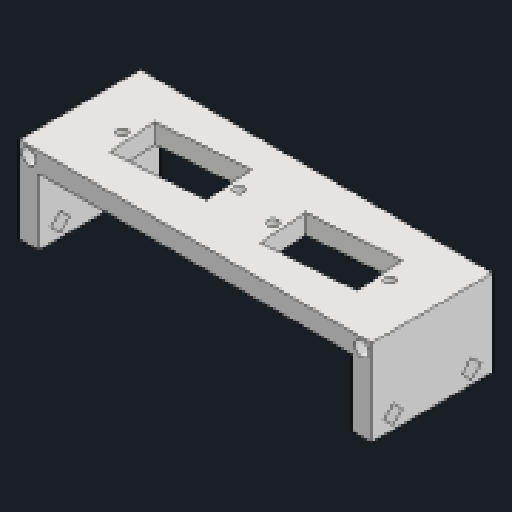
# Autodesk Inventor part: Module Frame
Saved by Autodesk Inventor 2023.2 (Build 272271030, 271C)
## iProperties
Created: 2024-02-26
Part Number: Module Frame
Material: Generic
Document SubType Name: Modeling
Designer: robpl
Density: 1 g/cm^3
Appearance: Default
Author: robpl
Autodesk Inventor part; units mm, degrees
ref_plane "YZ Plane" through (0, 0, 0) normal (1, 0, 0) x (0, 1, 0)
ref_plane "XZ Plane" through (0, 0, 0) normal (0, 1, 0) x (-1, 0, 0)
ref_plane "XY Plane" through (0, 0, 0) normal (0, 0, 1) x (1, 0, 0)
sketch "Sketch1" plane through (0, 0, 0) normal (0, 0, 1) x (1, 0, 0)
  line L0 (-40, 0) -> (40, 0)
  line L1 (40, 0) -> (40, 5)
  line L2 (40, 5) -> (-40, 5)
  line L3 (-40, 5) -> (-40, 0)
  line L4 (-40, 5) -> (-45, 5)
  line L5 (-45, 5) -> (-45, -17)
  line L6 (-45, -17) -> (-40, -17)
  line L7 (-40, -17) -> (-40, 5)
  line L8 (40, 5) -> (45, 5)
  line L9 (45, 5) -> (45, -17)
  line L10 (45, -17) -> (40, -17)
  line L11 (40, -17) -> (40, 5)
  point P0 (0, 0)
  point P1 (0, 0)
  point P2 (40, 0)
  dimension "d0" = 5
  dimension "d1" = 80
  dimension "d2" = 22
  dimension "d11" = 5
  constraints: 24 end point, 6 parallel, 3 horizontal, 3 perpendicular, 2 equal length, 1 coincident, 1 midpoint
  measures "d0" distance of L0.end L1.end
  measures "d1" distance of L0.start L0.end
  measures "d2" distance of L6.end L2.end
  measures "d11" distance of L9.end L10.end
extrude "Extrusion1" add sketch "Sketch1" along normal mid plane 31
sketch "Sketch2" plane through (45, -17, -15.5) normal (1, 0, 0) x (0, 0, -1)
  line L0 (-27.9042, 3.5) -> (-25.5, 1.0958)
  line L1 (-25.5, 1.0958) -> (-23.0958, 3.5)
  line L2 (-23.0958, 3.5) -> (-25.5, 5.9042)
  line L3 (-25.5, 5.9042) -> (-27.9042, 3.5)
  line L4 (-27.9042, 3.5) -> (-23.0958, 3.5) construction
  line L5 (-25.5, 1.0958) -> (-25.5, 5.9042) construction
  line L6 (-7.9042, 3.5) -> (-5.5, 1.0958)
  line L7 (-5.5, 1.0958) -> (-3.0958, 3.5)
  line L8 (-3.0958, 3.5) -> (-5.5, 5.9042)
  line L9 (-5.5, 5.9042) -> (-7.9042, 3.5)
  line L10 (-7.9042, 3.5) -> (-3.0958, 3.5) construction
  line L11 (-5.5, 1.0958) -> (-5.5, 5.9042) construction
  line L12 (0, 22) -> (-31, 22) projected
  point P0 (-15.5, 17)
  point P1 (-25.5, 3.5)
  point P2 (-5.5, 3.5)
  point P3 (-5.5, 3.5)
  point P4 (-25.5, 3.5)
  point P5 (-5.5, 3.5)
  point P6 (-15.5, 22)
  point P7 (-25.5, 3.5)
  dimension "d5" = 3.4
  dimension "d6" = 20
  dimension "d7" = 18.5
  dimension "d8" = 10
  constraints: 24 end point, 9 midpoint, 5 parallel, 5 perpendicular, 1 horizontal, 1 horizontal alignment
  measures "d5" distance of L0.end L1.end
  measures "d6" distance of point (-5.5, 3.5) point (-25.5, 3.5)
  measures "d7" distance from line of L12 point (-5.5, 3.5)
  measures "d8" horizontal distance of point (-15.5, 22) point (-25.5, 3.5)
extrude "Extrusion2" cut sketch "Sketch2" against normal through all
sketch "Sketch3" plane through (-45, 5, -15.5) normal (0, 1, 0) x (1, 0, 0)
  line L0 (39.1905, -14) -> (11.4768, -16.189)
  line L1 (50.8095, -17) -> (78.5232, -14.811)
  line L2 (0, 0) -> (90, 0) projected
  line L3 (0, 0) -> (0, -31) projected
  line L4 (90, -31) -> (0, -31) projected
  line L5 (90, 0) -> (90, -31) projected
  point P0 (45, -15.5)
  point P1 (69.8003, -15.5)
  point P2 (20.1997, -15.5)
  point P3 (90, -15.5)
  point P4 (45, -31)
  dimension "d12" = 12
  dimension "d13" = 27.8
  dimension "d14" = 19.05
  dimension "d15" = 19.05
  dimension "d16" = 31
  dimension "d17" = 11.6189
  dimension "d18" = 5.8095
  dimension "d19" = 3
  constraints: 4 end point, 2 horizontal alignment, 2 midpoint, 2 parallel, 2 point on line, 1 coincident
  measures "d12" distance of L0.start L1.start
  measures "d13" distance of L0.start L0.end
  measures "d14" distance of L1.start point (69.8, -15.5)
  measures "d15" distance of L0.start point (20.2, -15.5)
  measures "d16" distance of L2.end L4.start
  measures "d17" horizontal distance of L1.start L0.start
  measures "d18" horizontal distance of point (45, -31) L1.start
  measures "d19" vertical distance of L1.start L0.start
hole "Hole1" at (5.8095, 5, 1.5) at (-5.8095, 5, -1.5) at (33.5232, 5, -0.689) at (-33.5232, 5, 0.689) direction (0, -1, 0) diameter 2.5 end through all
sketch "Sketch4" plane through (-45, 5, -15.5) normal (0, 1, 0) x (1, 0, 0)
  circle A0 centre (78.5232, -14.811) radius 1.25 projected
  circle A1 centre (50.8095, -17) radius 1.25 projected
  circle A2 centre (39.1905, -14) radius 1.25 projected
  circle A3 centre (11.4768, -16.189) radius 1.25 projected
  line L0 (0, 0) -> (90, 0) projected
  line L1 (0, 0) -> (0, -31) projected
  line L2 (90, -31) -> (0, -31) projected
  line L3 (90, 0) -> (90, -31) projected
  circle A4 centre (50.8095, -17) radius 1.25 projected
  line L4 (78.5232, -14.811) -> (50.8095, -17)
  circle A5 centre (11.4768, -16.189) radius 1.25 projected
  line L5 (39.1905, -14) -> (11.4768, -16.189)
  line L6 (76.6227, -21.2306) -> (53.6941, -23.0416)
  line L7 (53.6941, -23.0416) -> (52.7099, -10.5804)
  line L8 (52.7099, -10.5804) -> (75.6385, -8.7694)
  line L9 (75.6385, -8.7694) -> (76.6227, -21.2306)
  line L10 (76.6227, -21.2306) -> (52.7099, -10.5804) construction
  line L11 (53.6941, -23.0416) -> (75.6385, -8.7694) construction
  line L12 (14.3615, -22.2306) -> (37.2901, -20.4196)
  line L13 (37.2901, -20.4196) -> (36.3059, -7.9584)
  line L14 (36.3059, -7.9584) -> (13.3773, -9.7694)
  line L15 (13.3773, -9.7694) -> (14.3615, -22.2306)
  line L16 (14.3615, -22.2306) -> (36.3059, -7.9584) construction
  line L17 (37.2901, -20.4196) -> (13.3773, -9.7694) construction
  point P0 (45, -15.5)
  point P1 (64.6663, -15.9055)
  point P2 (25.3337, -15.0945)
  point P3 (25.3337, -15.0945)
  dimension "d27" = 23
  dimension "d28" = 12.5
  constraints: 28 end point, 8 midpoint, 8 parallel, 2 perpendicular
  measures "d27" distance of L7.end L8.end
  measures "d28" distance of L6.end L7.end
extrude "Extrusion3" cut sketch "Sketch4" against normal through all contours L9 L6 L7 L4 | L4 L7 L8 L9 | L13 L12 L15 L5 | L5 L15 L14 L13
sketch "Sketch5" plane through (0, 0, -15.5) normal (0, 0, -1) x (-1, 0, 0)
  line L0 (-45, 5) -> (-45, -17) projected
  line L1 (-45, -17) -> (-40, -17) projected
  line L2 (-40, -17) -> (-40, 0) projected
  line L3 (-40, 0) -> (40, 0) projected
  line L4 (40, 0) -> (40, -17) projected
  line L5 (40, -17) -> (45, -17) projected
  line L6 (45, -17) -> (45, 5) projected
  line L7 (45, 5) -> (-45, 5) projected
  point P0 (0, 0)
  point P1 (-42.5, 2.5)
  point P2 (42.5, 2.5)
  dimension "d31" = 2.5
  dimension "d32" = 2.5
  dimension "d33" = 2.5
  constraints: 1 horizontal alignment
  measures "d31" distance from line of L0 point (-42.5, 2.5)
  measures "d32" distance from line of L7 point (-42.5, 2.5)
  measures "d33" distance from line of L6 point (42.5, 2.5)
hole "Hole2" at (42.5, 2.5, -15.5) at (-42.5, 2.5, -15.5) direction (0, 0, 1) diameter 3.7 depth 3.5
mirror "Mirror1" about plane through (0, 0, 0) normal (0, 0, 1) of "Hole2"
equation "\"d8\" = 0.5 * d6"
equation "\"d15\" = d14"
equation "\"d18\" = 0.5 * d17"
equation "\"d33\" = d31"
body "Solid1"
